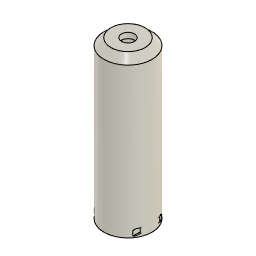
centra v3 (Autodesk Fusion 360 design; units mm, degrees)
Autodesk Fusion 360 part; units mm, degrees
sketch "Sketch1" plane through (0, 0, 0) normal (0, 0, 1) x (1, 0, 0)
  circle A0 centre (0, 0) radius 17.5
  circle A1 centre (0, 0) radius 12.5
  circle A2 centre (0, 0) radius 4.75
  dimension "d1" = 25
  dimension "d2" = 35
  dimension "d3" = 9.5
  constraint coincident A0.centre A1.centre
  constraint concentric A1 A2
  measures "d1" diameter of A1
  measures "d2" diameter of A0
  measures "d3" diameter of A2
extrude "Extrude1" add sketch "Sketch1" along normal blind 4 contours A0 | A1
extrude "Extrude2" add sketch "Sketch1" against normal blind 110 contours A0
chamfer "Chamfer1" distance 5 angle 45 1 edges at (-16.3157, -6.3283, 4)
chamfer "Chamfer2" distance 2 angle 45 1 edges at (-11.6541, -4.5202, -110)
sketch "Sketch2" plane through (0, 0, 0) normal (0, 1, 0) x (1, 0, 0)
  line L0 (0, 108.9485) -> (-12.5, 108.9485)
  line L1 (0, 108.9485) -> (12.5, 108.9485)
  line L2 (-16, 108.9485) -> (-14, 108.9485)
  line L3 (-14, 108.9485) -> (-14, 104.4591)
  line L4 (-14, 104.4591) -> (-16, 104.4591)
  line L5 (-16, 104.4591) -> (-16, 108.9485)
  line L6 (14, 104.4591) -> (16, 104.4591)
  line L7 (16, 104.4591) -> (16, 108.9485)
  line L8 (16, 108.9485) -> (14, 108.9485)
  line L9 (14, 108.9485) -> (14, 104.4591)
  line L10 (-15, 118.4485) -> (-15, 99.4485)
  line L11 (15, 119.4485) -> (15, 98.4485)
  line L12 (-12.5, 108.9485) -> (-17.5, 108.9485)
  line L13 (12.5, 108.9485) -> (17.5, 108.9485)
  dimension "d10" = 12.5
  dimension "d11" = 12.5
  dimension "d12" = 2
  dimension "d13" = 2
  dimension "d14" = 5
  dimension "d15" = 5
  constraint horizontal L0
  constraint parallel L0 L1
  constraint horizontal L2
  constraint vertical L3
  constraint horizontal L4
  constraint vertical L5
  constraint horizontal L6
  constraint vertical L7
  constraint horizontal L8
  constraint vertical L9
  constraint equal L3 L9
  constraint vertical L10
  constraint vertical L11
  constraint midpoint L2 L10
  constraint parallel L0 L12
  constraint perpendicular L11 L13
  constraint midpoint L11 L13
  constraint midpoint L10 L12
  constraint midpoint L8 L11
  measures "d10" distance of L0.start L0.end
  measures "d11" distance of L0.start L1.end
  measures "d12" distance of L2.start L2.end
  measures "d13" distance of L6.start L6.end
  measures "d14" distance of L1.end L13.end
  measures "d15" distance of L0.end L12.end
extrude "Extrude3" cut sketch "Sketch2" along normal blind 100
extrude "Extrude4" cut 2 faces at (14.6667, 0, -107.452) (-15.3333, 0, -107.452) along direction (0, -1, 0) blind 100
chamfer "Chamfer3" distance 1 angle 45 4 edges at (14, 0, -104.4591) (-14, 0, -104.4591) (16, 0, -108.9485) (-16, 0, -108.9485)
equation "d10 = ( 25 / 2 ) * 1 mm"
